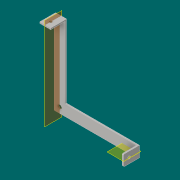
# Autodesk Inventor part: Ell-Tab
Saved by Autodesk Inventor 2016 (Build 200138000, 138)
## iProperties
Created: 2017-01-14
Part Number: Ell-Tab
Material: Generic
Document SubType Name: Modeling
Designer: katzchristy
Density: 1 g/cm^3
Appearance: Default
Author: katzchristy
Autodesk Inventor part; units mm, degrees
ref_plane "YZ Plane" through (0, 0, 0) normal (1, 0, 0) x (0, 1, 0)
ref_plane "XZ Plane" through (0, 0, 0) normal (0, 1, 0) x (-1, 0, 0)
ref_plane "XY Plane" through (0, 0, 0) normal (0, 0, 1) x (1, 0, 0)
sketch "Sketch1" plane through (0, 0, 0) normal (1, 0, 0) x (0, 1, 0)
  line L0 (70.1502, -64.6199) -> (54.9102, -64.6199)
  line L1 (54.9102, -64.6199) -> (54.9102, -42.5219)
  line L2 (54.9102, -42.5219) -> (70.1502, -42.5219)
  line L3 (70.1502, -42.5219) -> (70.1502, -64.6199)
  point P0 (0, 0)
  dimension "d0" = 22.098
  dimension "d1" = 15.24
  constraints: 8 end point, 2 parallel, 1 horizontal, 1 perpendicular
  measures "d0" distance of L0.end L1.end
  measures "d1" distance of L0.start L0.end
extrude "Extrusion1" add sketch "Sketch1" against normal blind 2.032
sketch "Sketch2" plane through (-2.032, 0, 0) normal (-1, 0, 0) x (0, 0, 1)
  line L0 (-64.6199, 54.9102) -> (-62.5879, 54.9102)
  line L1 (-62.5879, 54.9102) -> (-62.5879, 70.1502)
  line L2 (-62.5879, 70.1502) -> (-64.6199, 70.1502)
  line L3 (-64.6199, 70.1502) -> (-64.6199, 54.9102)
  line L4 (-64.6199, 70.1502) -> (-64.6199, 54.9102) projected
  line L5 (-42.5219, 70.1502) -> (-64.6199, 70.1502) projected
  line L6 (-64.6199, 54.9102) -> (-42.5219, 54.9102) projected
  point P0 (0, 0)
  dimension "d4" = 2.032
  constraints: 8 end point, 3 collinear, 2 parallel, 1 horizontal, 1 perpendicular
  measures "d4" distance of L1.end L2.end
extrude "Extrusion2" add sketch "Sketch2" along normal blind 19.05
sketch "Sketch3" plane through (0, 0, 0) normal (1, 0, 0) x (0, 0, -1)
  circle A0 centre (50.1419, 62.5302) radius 2.032
  line L0 (42.5219, 54.9102) -> (42.5219, 70.1502) projected
  point P0 (0, 0)
  point P1 (42.5219, 62.5302)
  dimension "d7" = 7.62
  dimension "d8" = 4.064
  constraints: 1 centre point, 1 horizontal alignment, 1 midpoint
  measures "d7" distance from line of L0 A0.centre
  measures "d8" diameter of A0
extrude "Extrusion3" cut sketch "Sketch3" against normal up to next
fillet "Fillet1" radius 1.27 2 edges at (-1.016, 54.9102, -42.5219) (-1.016, 70.1502, -42.5219)
ref_plane "Work Plane1" through (-21.082, 62.5302, -64.6199) normal (0, 1, 0) x (1, 0, 0)
sketch "Sketch4" plane through (-2.032, 54.9102, -62.5879) normal (0, 0, 1) x (1, 0, 0)
  line L0 (0, 0) -> (-19.05, 0) projected
  line L1 (-19.05, 0) -> (-114.808, 0)
  line L2 (-114.808, 0) -> (-114.808, 95.758)
  line L3 (-114.808, 95.758) -> (-99.568, 95.758)
  line L4 (-99.568, 95.758) -> (-99.568, 15.24)
  line L5 (0, 15.24) -> (-19.05, 15.24) projected
  line L6 (-99.568, 15.24) -> (-19.05, 15.24)
  line L7 (-19.05, 15.24) -> (-19.05, 0)
  circle A0 centre (-107.188, 7.62) radius 3.175
  line L8 (2.032, 1.27) -> (2.032, 13.97) projected
  point P0 (2.032, -54.9102)
  point P1 (-107.188, 95.758)
  dimension "d12" = 6.35
  dimension "d13" = 15.24
  dimension "d14" = 109.22
  dimension "d15" = 88.138
  constraints: 12 end point, 3 perpendicular, 2 horizontal, 1 centre point, 1 midpoint, 1 parallel, 1 vertical alignment
  measures "d12" diameter of A0
  measures "d13" distance of L2.end L3.end
  measures "d14" distance from line of L8 A0.centre
  measures "d15" distance from line of L3 A0.centre
extrude "Extrusion4" add sketch "Sketch4" against normal up to surface (2.032 mm away)
pattern_circular "Circular Pattern1" count 2 over 90 about axis through (-109.22, 62.5302, -62.5879) along (0, 0, 1) of "Extrusion2", "Extrusion1", "Extrusion3"
ref_plane "Work Plane2" through (-109.22, 169.7182, -62.5879) normal (-1, 0, 0) x (0, 0, 1)
body "Solid1"
